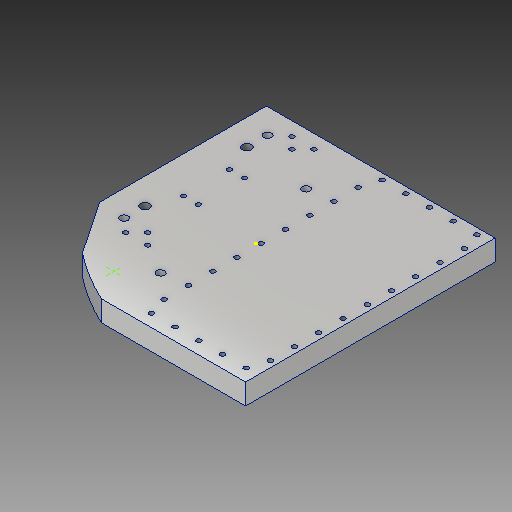
# Autodesk Inventor part: Base Plate Mk 2
Saved by Autodesk Inventor 2017 (Build 210142000, 142)
## iProperties
Created: 2016-12-06
Part Number: Base Plate Mk 2
Material: Aluminum 6061
Document SubType Name: Modeling
Designer: qupec
Density: 2.7 g/cm^3
Appearance: Aluminum - Flat
Mass: 681.535 g
Surface Area: 529.714 cm^2
Volume: 252.42 cm^3
Author: qupec
Autodesk Inventor part; units mm, degrees
ref_plane "YZ Plane" through (0, 0, 0) normal (1, 0, 0) x (0, 1, 0)
ref_plane "XZ Plane" through (0, 0, 0) normal (0, 1, 0) x (-1, 0, 0)
ref_plane "XY Plane" through (0, 0, 0) normal (0, 0, 1) x (1, 0, 0)
sketch "Sketch1" plane through (0, 0, 0) normal (0, 1, 0) x (-1, 0, 0)
  line L0 (69.85, 76.2) -> (-69.85, 76.2)
  line L1 (-69.85, 76.2) -> (-69.85, -76.2)
  line L2 (-69.85, -76.2) -> (69.85, -76.2)
  line L3 (69.85, -76.2) -> (69.85, 76.2)
  point P0 (0, 0)
  dimension "d0" = 152.4
  dimension "d1" = 139.7
  dimension "d2" = 69.85
  dimension "d3" = 76.2
  constraints: 8 end point, 2 parallel, 1 horizontal, 1 perpendicular
  measures "d0" distance of L2.end L0.start
  measures "d1" distance of L0.start L0.end
  measures "d2" distance from line of point (0, 0) L1
  measures "d3" distance from line of point (0, 0) L0
extrude "Extrusion1" add sketch "Sketch1" along normal blind 12.7
sketch "Sketch4" plane through (0, 12.7, 0) normal (0, 1, 0) x (1, 0, 0)
  circle A0 centre (63.5, 69.85) radius 3.175
  circle A1 centre (63.5, -69.85) radius 3.175
  circle A2 centre (-60.96, -52.07) radius 3.175
  line L0 (69.85, 76.2) -> (-69.85, 76.2) projected
  line L1 (69.85, -76.2) -> (69.85, 76.2) projected
  line L2 (-69.85, -76.2) -> (69.85, -76.2) projected
  line L3 (-69.85, 76.2) -> (-69.85, -76.2) projected
  circle A3 centre (-60.96, 52.07) radius 3.175
  point P0 (0, 0)
  dimension "d20" = 6.35
  dimension "d21" = 6.35
  dimension "d22" = 6.35
  dimension "d23" = 6.35
  dimension "d24" = 6.35
  dimension "d25" = 6.35
  dimension "d26" = 6.35
  dimension "d27" = 24.13
  dimension "d28" = 8.89
  dimension "d32" = 6.35
  dimension "d33" = 24.13
  dimension "d34" = 8.89
  constraints: 4 centre point
  measures "d20" diameter of A2
  measures "d21" diameter of A1
  measures "d22" diameter of A0
  measures "d23" distance from line of L0 A0.centre
  measures "d24" distance from line of L1 A0.centre
  measures "d25" distance from line of L1 A1.centre
  measures "d26" distance from line of L2 A1.centre
  measures "d27" distance from line of L2 A2.centre
  measures "d28" distance from line of L3 A2.centre
  measures "d32" diameter of A3
  measures "d33" distance from line of L0 A3.centre
  measures "d34" distance from line of L3 A3.centre
extrude "Extrusion6" [suppressed]
fillet "Fillet1" [suppressed]
sketch "Sketch7" plane through (0, 12.7, 0) normal (0, 1, 0) x (1, 0, 0)
  arc A0 (-69.85, -37.0366) -> (-18.2851, -76.2) centre (46.0045, 61.976) ccw
  line L0 (69.85, 76.2) -> (-69.85, 76.2) projected
  line L1 (69.85, -76.2) -> (69.85, 76.2) projected
  line L2 (-69.85, 76.2) -> (-69.85, -76.2) projected
  line L3 (-69.85, -76.2) -> (69.85, -76.2) projected
  line L4 (-69.85, 76.2) -> (-69.85, -76.2) projected
  arc A1 (-18.2851, -76.2) -> (-69.85, -37.0366) centre (46.0045, 61.976) ccw
  point P0 (0, 0)
  point P1 (76.2, -60.325)
  point P2 (73.025, -60.325)
  point P3 (73.025, 63.5)
  point P4 (73.025, 60.325)
  point P5 (-73.025, 63.5)
  point P6 (76.2, 60.325)
  point P7 (73.025, -63.5)
  point P8 (-76.2, 60.325)
  point P9 (-80.9955, -22.2663)
  dimension "d46" = 304.8
  dimension "d47" = 14.224
  dimension "d48" = 23.8455
  constraints: 5 point on circle, 2 centre point, 7 other
  measures "d46" diameter of A0
sketch "Sketch8" plane through (0, 12.7, 0) normal (0, 1, 0) x (1, 0, 0)
  circle A0 centre (-32.4275, -33.782) radius 1.4224 projected
  circle A1 centre (-39.1585, -27.051) radius 1.4224 projected
  circle A2 centre (-45.8895, -33.782) radius 1.4224 projected
  circle A3 centre (-45.8895, 67.818) radius 1.4224 projected
  circle A4 centre (-39.1585, 61.087) radius 1.4224 projected
  circle A5 centre (-32.4275, 67.818) radius 1.4224 projected
  circle A6 centre (-47.526, 3.308) radius 1.4224 projected
  circle A7 centre (-47.526, 3.308) radius 1.4224 projected
  circle A8 centre (-38.506, 3.308) radius 1.4224 projected
  line L0 (-33.996, 0.7903) -> (-52.036, 0.7903) projected
  line L1 (-33.996, 5.8258) -> (-33.996, 0.7903) projected
  line L2 (-33.996, 5.8258) -> (-52.036, 5.8258) projected
  line L3 (-52.036, 0.7903) -> (-52.036, 5.8258) projected
  circle A9 centre (-47.526, 31.2925) radius 1.4224 projected
  circle A10 centre (-38.506, 31.2925) radius 1.4224 projected
  line L4 (-33.996, 28.7747) -> (-52.036, 28.7747) projected
  line L5 (-33.996, 33.8103) -> (-33.996, 28.7747) projected
  line L6 (-33.996, 33.8103) -> (-52.036, 33.8103) projected
  line L7 (-52.036, 28.7747) -> (-52.036, 33.8103) projected
  circle A11 centre (2.54, -39.6875) radius 3.175 construction
  circle A12 centre (2.54, 12.7127) radius 3.175 construction
  circle A13 centre (2.54, 65.1129) radius 3.175 construction
  circle A14 centre (68.58, 65.1129) radius 3.175 construction
  circle A15 centre (68.58, 12.7127) radius 3.175 construction
  circle A16 centre (68.58, -39.6875) radius 3.175 construction
extrude "Extrusion9" cut sketch "Sketch8" against normal through all contours A0 | A1 | A2 | A3 | A4 | A5 | A6 | A8 | A9 | A10
extrude "Extrusion11" cut sketch "Sketch7" against normal through all contours A0 L3 L2
sketch "Sketch10" plane through (0, 12.7, 0) normal (0, 1, 0) x (1, 0, 0)
  circle A0 centre (62.611, 72.39) radius 1.4732 projected
  arc A1 (-69.85, -37.0366) -> (-18.2851, -76.2) centre (46.0045, 61.976) ccw projected
  line L0 (-18.2851, -76.2) -> (69.85, -76.2) projected
  line L1 (69.85, -76.2) -> (69.85, 76.2) projected
  line L2 (69.85, 76.2) -> (-69.85, 76.2) projected
  line L3 (-69.85, 76.2) -> (-69.85, -37.0366) projected
  circle A2 centre (-47.526, 31.2925) radius 1.4224 projected
  circle A3 centre (-47.526, 3.308) radius 1.4224 projected
  circle A4 centre (-39.1585, 61.087) radius 1.4224 projected
  circle A5 centre (-45.8895, -33.782) radius 1.4224 projected
  circle A6 centre (-32.4275, -33.782) radius 1.4224 projected
  circle A7 centre (-39.1585, -27.051) radius 1.4224 projected
  circle A8 centre (-45.8895, 67.818) radius 1.4224 projected
  circle A9 centre (-32.4275, 67.818) radius 1.4224 projected
  circle A10 centre (-38.506, 3.308) radius 1.4224 projected
  circle A11 centre (-38.506, 31.2925) radius 1.4224 projected
  circle A12 centre (33.655, 72.39) radius 1.4732 projected
  circle A13 centre (48.133, 72.39) radius 1.4732 projected
  circle A14 centre (19.177, 72.39) radius 1.4732 projected
  circle A15 centre (4.699, 72.39) radius 1.4732 projected
  circle A16 centre (62.611, -68.58) radius 1.4732 projected
  circle A17 centre (48.133, -68.58) radius 1.4732 projected
  circle A18 centre (33.655, -68.58) radius 1.4732 projected
  circle A19 centre (19.177, -68.58) radius 1.4732 projected
  circle A20 centre (4.699, -68.58) radius 1.4732 projected
  point P0 (0, 0)
extrude "Extrusion13" cut sketch "Sketch10" against normal through all contours A0 | A12 | A13 | A14 | A15 | A16 | A17 | A18 | A19 | A20
sketch "Sketch11" plane through (0, 12.7, 0) normal (0, 1, 0) x (1, 0, 0)
  circle A0 centre (19.177, 72.39) radius 1.4732 projected
  circle A1 centre (48.133, 72.39) radius 1.4732 projected
  circle A2 centre (62.611, -68.58) radius 1.4732 projected
  circle A3 centre (33.655, -68.58) radius 1.4732 projected
  circle A4 centre (4.699, -68.58) radius 1.4732 projected
  circle A5 centre (1.27, -42.545) radius 1.4732 projected
  circle A6 centre (1.27, -12.9117) radius 1.4732 projected
  circle A7 centre (1.27, 16.7217) radius 1.4732 projected
  circle A8 centre (1.27, 46.355) radius 1.4732 projected
  circle A9 centre (66.04, 61.1717) radius 1.4732 projected
  circle A10 centre (66.04, 31.5383) radius 1.4732 projected
  circle A11 centre (66.04, 1.905) radius 1.4732 projected
  circle A12 centre (66.04, -27.7283) radius 1.4732 projected
  circle A13 centre (66.04, -57.3617) radius 1.4732 projected
  circle A14 centre (66.04, -42.545) radius 1.4732 projected
  circle A15 centre (66.04, -12.9117) radius 1.4732 projected
  circle A16 centre (66.04, 16.7217) radius 1.4732 projected
  circle A17 centre (66.04, 46.355) radius 1.4732 projected
  circle A18 centre (1.27, 61.1717) radius 1.4732 projected
  circle A19 centre (1.27, 31.5383) radius 1.4732 projected
  circle A20 centre (1.27, 1.905) radius 1.4732 projected
  circle A21 centre (1.27, -27.7283) radius 1.4732 projected
  circle A22 centre (1.27, -57.3617) radius 1.4732 projected
  circle A23 centre (19.177, -68.58) radius 1.4732 projected
  circle A24 centre (48.133, -68.58) radius 1.4732 projected
  circle A25 centre (62.611, 72.39) radius 1.4732 projected
  circle A26 centre (33.655, 72.39) radius 1.4732 projected
  circle A27 centre (4.699, 72.39) radius 1.4732 projected
  line L0 (0.635, -72.39) -> (66.675, -72.39) projected
  line L1 (69.85, -69.215) -> (69.85, 73.025) projected
  line L2 (66.675, 76.2) -> (0.635, 76.2) projected
  line L3 (-2.54, 73.025) -> (-2.54, -69.215) projected
  arc A28 (59.055, 62.23) -> (55.88, 65.405) centre (55.88, 62.23) ccw projected
  line L4 (59.055, -58.42) -> (59.055, 62.23) projected
  arc A29 (55.88, -61.595) -> (59.055, -58.42) centre (55.88, -58.42) ccw projected
  line L5 (11.43, -61.595) -> (55.88, -61.595) projected
  arc A30 (8.255, -58.42) -> (11.43, -61.595) centre (11.43, -58.42) ccw projected
  line L6 (8.255, 62.23) -> (8.255, -58.42) projected
  arc A31 (11.43, 65.405) -> (8.255, 62.23) centre (11.43, 62.23) ccw projected
  line L7 (55.88, 65.405) -> (11.43, 65.405) projected
  arc A32 (69.85, 73.025) -> (66.675, 76.2) centre (66.675, 73.025) ccw projected
  arc A33 (0.635, 76.2) -> (-2.54, 73.025) centre (0.635, 73.025) ccw projected
  arc A34 (-2.54, -69.215) -> (0.635, -72.39) centre (0.635, -69.215) ccw projected
  arc A35 (66.675, -72.39) -> (69.85, -69.215) centre (66.675, -69.215) ccw projected
  point P0 (0, 0)
  point P1 (52.705, -61.595)
extrude "Extrusion14" cut sketch "Sketch11" against normal through all contours A5 | A6 | A7 | A8 | A9 | A10 | A11 | A12 | A13 | A14 | A15 | A16 | A17 | A18 | A19 | A20 | A21 | A22 | A25
sketch "Sketch12" plane through (0, 12.7, 0) normal (0, 1, 0) x (1, 0, 0)
  line L0 (-69.85, 76.2) -> (-69.85, -37.0366) projected
  line L1 (69.85, 76.2) -> (-69.85, 76.2) projected
  circle A0 centre (-47.526, 31.2925) radius 1.4224 projected
  circle A1 centre (-47.526, 3.308) radius 1.4224 projected
  line L2 (-47.526, 17.3003) -> (-38.0708, 17.3003) construction
  point P0 (0, 0)
  point P1 (-53.975, -13.8147)
  point P2 (-53.975, 48.4153)
  dimension "d63" = 15.875
  dimension "d64" = 15.875
  dimension "d75" = 13.9922
  dimension "d76" = 27.9845
  dimension "d77" = 31.115
  dimension "d78" = 31.115
  constraints: 2 end point, 1 horizontal
  measures "d63" distance from line of L0 point (-53.975, 48.415)
  measures "d64" distance from line of L0 point (-53.975, -13.815)
  measures "d75" distance from line of A1.centre L2
  measures "d76" distance of A0.centre A1.centre
  measures "d77" distance from line of L2 point (-53.975, -13.815)
  measures "d78" distance from line of L2 point (-53.975, 48.415)
hole "Hole1" at (-53.975, 12.7, 13.8147) at (-53.975, 12.7, -48.4153) direction (0, -1, 0) diameter 5.588 depth 25.4 tip angle 118
sketch "Sketch14" plane through (0, 0, 0) normal (0, -1, 0) x (1, 0, 0)
  line L0 (69.85, -76.2) -> (-69.85, -76.2) projected
  line L1 (-18.2851, 76.2) -> (69.85, 76.2) projected
  circle A0 centre (4.699, -72.39) radius 1.4732 projected
  circle A1 centre (-32.4275, -67.818) radius 1.4224 projected
  point P0 (0, 0)
  point P1 (-13.8642, 44.45)
  point P2 (-13.8642, -44.45)
  dimension "d79" = 44.45
  dimension "d80" = 152.4
  dimension "d81" = 44.45
  dimension "d82" = 37.1265
  dimension "d83" = 18.5633
  dimension "d84" = 18.5633
  measures "d79" vertical distance of point (0, 0) point (-13.864, 44.45)
  measures "d80" distance between parallel lines of L0 L1
  measures "d81" vertical distance of point (-13.864, -44.45) point (0, 0)
  measures "d82" horizontal distance of A0.centre A1.centre
  measures "d83" horizontal distance of A1.centre point (-13.864, -44.45)
  measures "d84" horizontal distance of A1.centre point (-13.864, 44.45)
hole "Hole2" at (-13.8642, 0, 44.45) at (-13.8642, 0, -44.45) direction (0, 1, 0) diameter 4.826 depth 12.7 tip angle 118
sketch "Sketch15" plane through (0, 0, 0) normal (0, -1, 0) x (1, 0, 0)
  circle A0 centre (-13.8642, 44.45) radius 2.413 projected
  circle A1 centre (-13.8642, -44.45) radius 2.413 projected
  circle A2 centre (66.04, -31.5383) radius 1.4732 projected
  circle A3 centre (1.27, -31.5383) radius 1.4732 projected
  circle A4 centre (1.27, 42.545) radius 1.4732 projected
  point P0 (0, 0)
  point P1 (33.655, -44.45)
  point P2 (33.655, 44.45)
  point P3 (33.655, 0)
  dimension "d92" = 44.45
  dimension "d93" = 44.45
  dimension "d94" = 44.45
  dimension "d95" = 44.45
  dimension "d96" = 64.77
  dimension "d97" = 32.385
  dimension "d98" = 32.385
  dimension "d222" = 32.385
  dimension "d223" = 44.45
  measures "d92" vertical distance of point (0, 0) point (33.655, 44.45)
  measures "d93" vertical distance of point (0, 0) A0.centre
  measures "d94" vertical distance of point (0, 0) A1.centre
  measures "d95" vertical distance of point (33.655, -44.45) point (0, 0)
  measures "d96" distance between centres of A2 A3
  measures "d97" horizontal distance of A3.centre point (33.655, -44.45)
  measures "d98" horizontal distance of point (33.655, 44.45) A4.centre
  measures "d222" horizontal distance of A4.centre point (33.655, 0)
  measures "d223" distance of point (33.655, -44.45) point (33.655, 0)
hole "Hole3" at (33.655, 0, -44.45) at (33.655, 0, 44.45) at (33.655, 0, 0) direction (0, 1, 0) diameter 4.826 depth 9.525
thread "Thread3" size "5-40 UNC" class "2B" standard "ANSI Unified Screw Threads" full length
thread "Thread4" size "5-40 UNC" class "2B" standard "ANSI Unified Screw Threads" full length
thread "Thread5" size "5-40 UNC" class "2B" standard "ANSI Unified Screw Threads" full length
thread "Thread6" size "5-40 UNC" class "2B" standard "ANSI Unified Screw Threads" full length
thread "Thread7" size "5-40 UNC" class "2B" standard "ANSI Unified Screw Threads" full length
thread "Thread8" size "5-40 UNC" class "2B" standard "ANSI Unified Screw Threads" full length
thread "Thread9" size "5-40 UNC" class "2B" standard "ANSI Unified Screw Threads" full length
thread "Thread10" size "5-40 UNC" class "2B" standard "ANSI Unified Screw Threads" full length
thread "Thread11" size "5-40 UNC" class "2B" standard "ANSI Unified Screw Threads" full length
thread "Thread12" size "5-40 UNC" class "2B" standard "ANSI Unified Screw Threads" full length
thread "Thread13" size "5-40 UNC" class "2B" standard "ANSI Unified Screw Threads" full length
thread "Thread14" size "5-40 UNC" class "2B" standard "ANSI Unified Screw Threads" full length
thread "Thread15" size "5-40 UNC" class "2B" standard "ANSI Unified Screw Threads" full length
thread "Thread16" size "5-40 UNC" class "2B" standard "ANSI Unified Screw Threads" full length
thread "Thread17" size "5-40 UNC" class "2B" standard "ANSI Unified Screw Threads" full length
thread "Thread18" size "5-40 UNC" class "2B" standard "ANSI Unified Screw Threads" full length
thread "Thread19" size "5-40 UNC" class "2B" standard "ANSI Unified Screw Threads" full length
thread "Thread20" size "5-40 UNC" class "2B" standard "ANSI Unified Screw Threads" full length
thread "Thread21" size "5-40 UNC" class "2B" standard "ANSI Unified Screw Threads" full length
thread "Thread22" size "5-40 UNC" class "2B" standard "ANSI Unified Screw Threads" full length
thread "Thread23" size "5-40 UNC" class "2B" standard "ANSI Unified Screw Threads" full length
thread "Thread24" size "5-40 UNC" class "2B" standard "ANSI Unified Screw Threads" full length
thread "Thread25" size "5-40 UNC" class "2B" standard "ANSI Unified Screw Threads" full length
thread "Thread26" size "5-40 UNC" class "2B" standard "ANSI Unified Screw Threads" full length
thread "Thread27" size "5-40 UNC" class "2B" standard "ANSI Unified Screw Threads" full length
thread "Thread28" size "5-40 UNC" class "2B" standard "ANSI Unified Screw Threads" full length
thread "Thread29" size "5-40 UNC" class "2B" standard "ANSI Unified Screw Threads" full length
thread "Thread30" size "5-40 UNC" class "2B" standard "ANSI Unified Screw Threads" full length
thread "Thread31" size "5-40 UNC" class "2B" standard "ANSI Unified Screw Threads" full length
thread "Thread32" size "4-40 UNC" class "2B" standard "ANSI Unified Screw Threads" full length
thread "Thread33" size "4-40 UNC" class "2B" standard "ANSI Unified Screw Threads" full length
thread "Thread34" size "4-40 UNC" class "2B" standard "ANSI Unified Screw Threads" full length
thread "Thread35" size "4-40 UNC" class "2B" standard "ANSI Unified Screw Threads" full length
thread "Thread36" size "4-40 UNC" class "2B" standard "ANSI Unified Screw Threads" full length
thread "Thread37" size "4-40 UNC" class "2B" standard "ANSI Unified Screw Threads" full length
thread "Thread38" size "4-40 UNC" class "2B" standard "ANSI Unified Screw Threads" full length
thread "Thread39" size "4-40 UNC" class "2B" standard "ANSI Unified Screw Threads" full length
thread "Thread40" size "4-40 UNC" class "2B" standard "ANSI Unified Screw Threads" full length
thread "Thread41" size "4-40 UNC" class "2B" standard "ANSI Unified Screw Threads" full length
thread "Thread42" size "1/4-20 UNC" class "2B" standard "ANSI Unified Screw Threads" full length
thread "Thread43" size "1/4-20 UNC" class "2B" standard "ANSI Unified Screw Threads" full length
sketch "Sketch16" plane through (0, 0, 0) normal (0, -1, 0) x (1, 0, 0)
  line L0 (-18.2851, 76.2) -> (69.85, 76.2) projected
  line L1 (69.85, -76.2) -> (-69.85, -76.2) projected
  line L2 (69.85, 76.2) -> (63.5, 76.2)
  line L3 (63.5, 76.2) -> (63.5, -76.2)
  line L4 (63.5, -76.2) -> (69.85, -76.2)
  line L5 (69.85, -76.2) -> (69.85, 76.2)
  point P0 (0, 0)
  dimension "d196" = 6.35
  constraints: 8 end point, 2 parallel, 1 horizontal, 1 perpendicular, 1 point on line
  measures "d196" distance of L4.end L3.end
extrude "Extrusion15" [suppressed]
sketch "Sketch17" plane through (0, 12.7, 0) normal (0, 1, 0) x (1, 0, 0)
  line L0 (-48.26, -57.7736) -> (-69.85, -25.6538)
  line L1 (-69.85, 76.2) -> (-69.85, -37.0366) projected
  line L2 (-69.85, -25.6538) -> (-69.85, -37.0366)
  arc A0 (-69.85, -37.0366) -> (-18.2851, -76.2) centre (46.0045, 61.976) ccw projected
  arc A1 (-69.85, -37.0366) -> (-48.26, -57.7736) centre (46.0045, 61.976) ccw
  point P0 (0, 0)
  dimension "d200" = 6.35
  dimension "d203" = 21.59
  constraints: 4 end point, 3 point on circle, 1 centre point, 1 concentric, 1 point on line
  measures "d200" distance from line of L1.end L0
  measures "d203" horizontal distance of L1.end L0.start
extrude "Extrusion16" cut sketch "Sketch17" against normal through all
thread "Thread46" size "10-32 UNF" class "2B" standard "ANSI Unified Screw Threads" full length
thread "Thread47" size "10-32 UNF" class "2B" standard "ANSI Unified Screw Threads" full length
thread "Thread48" size "10-32 UNF" class "2B" standard "ANSI Unified Screw Threads" full length
sketch "Sketch18" plane through (0, 12.7, 0) normal (0, 1, 0) x (1, 0, 0)
  circle A0 centre (-53.975, -13.8147) radius 2.794 projected
  circle A1 centre (-53.975, 48.4153) radius 2.794 projected
  point P0 (0, 0)
  point P1 (-53.975, 61.1153)
  point P2 (-53.975, -26.5147)
  dimension "d211" = 12.7
  dimension "d212" = 12.7
  dimension "d213" = 0
  dimension "d214" = 0
  measures "d211" distance of A0.centre point (-53.975, -26.515)
  measures "d212" distance of A1.centre point (-53.975, 61.115)
  measures "d213" horizontal distance of A1.centre point (-53.975, 61.115)
  measures "d214" horizontal distance of A0.centre point (-53.975, -26.515)
hole "Hole4" at (-53.975, 12.7, -61.1153) at (-53.975, 12.7, 26.5147) direction (0, -1, 0) diameter 4.826 depth 12.7
sketch "Sketch19" plane through (0, 12.7, 0) normal (0, 1, 0) x (1, 0, 0)
  point P0 (0, 0)
  point P1 (-28.9602, -57.9611)
equation "\"d2\" = 0.5 * d1"
equation "\"d3\" = 0.5 * d0"
equation "\"d21\" = d20"
equation "\"d22\" = d20"
equation "\"d24\" = d23"
equation "\"d25\" = d24"
equation "\"d26\" = d23"
equation "\"d32\" = d20"
equation "\"d33\" = d27"
equation "\"d34\" = d28"
equation "\"d63\" = d64"
equation "\"d75\" = 0.5 * d76"
equation "\"d78\" = d77"
equation "\"d79\" = d81"
equation "\"d83\" = 0.5 * d82"
equation "\"d84\" = d83"
equation "\"d92\" = d93"
equation "\"d95\" = d94"
equation "\"d97\" = 0.5 * d96"
equation "\"d98\" = d97"
equation "\"d222\" = d98"
equation "\"d223\" = d95"
body "Solid1"
